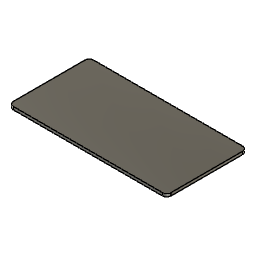
ESP 32 Lid v0 (Autodesk Fusion 360 design; units mm, degrees)
Autodesk Fusion 360 part; units mm, degrees
sketch "Sketch1" plane through (0, 0, 0) normal (0, 0, 1) x (1, 0, 0)
  line L0 (1.5, 0) -> (53.5, 0)
  line L1 (55, 1.5) -> (55, 26.5)
  line L2 (53.5, 28) -> (1.5, 28)
  line L3 (0, 26.5) -> (0, 1.5)
  arc A0 (55, 26.5) -> (53.5, 28) centre (53.5, 26.5) ccw
  arc A1 (53.5, 0) -> (55, 1.5) centre (53.5, 1.5) ccw
  arc A2 (1.5, 28) -> (0, 26.5) centre (1.5, 26.5) ccw
  arc A3 (0, 1.5) -> (1.5, 0) centre (1.5, 1.5) ccw
  point P0 (55, 28)
  point P1 (0, 28)
  dimension "d1" = 28
  dimension "d2" = 55
  dimension "d3" = 1.5
  dimension "d4" = 1.5
  dimension "d5" = 1.5
  dimension "d6" = 1.5
  constraint horizontal L0
  constraint vertical L1
  constraint horizontal L2
  constraint vertical L3
  constraint coincident P0 L1
  constraint coincident P0 L2
  constraint tangent L1 A0
  constraint tangent L2 A0
  constraint tangent L1 A1
  constraint tangent L0 A1
  constraint coincident P1 L2
  constraint coincident P1 L3
  constraint tangent L2 A2
  constraint tangent L3 A2
  constraint coincident origin L3
  constraint coincident origin L0
  constraint tangent L3 A3
  constraint tangent L0 A3
  measures "d1" distance of origin P1
  measures "d2" distance of P0 P1
  measures "d3" radius of A0
  measures "d4" radius of A1
  measures "d5" radius of A2
  measures "d6" radius of A3
extrude "Extrude1" add sketch "Sketch1" along normal blind 1
